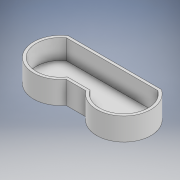
# Autodesk Inventor part: paitent remote box
Saved by Autodesk Inventor 2021 (Build 250183000, 183)
## iProperties
Created: 2023-01-12
Part Number: paitent remote box
Material: Generic
Document SubType Name: Modeling
Designer: boyle
Density: 1 g/cm^3
Appearance: Default
Author: boyle
Autodesk Inventor part; units mm, degrees
ref_plane "YZ Plane" through (0, 0, 0) normal (1, 0, 0) x (0, 1, 0)
ref_plane "XZ Plane" through (0, 0, 0) normal (0, 1, 0) x (-1, 0, 0)
ref_plane "XY Plane" through (0, 0, 0) normal (0, 0, 1) x (1, 0, 0)
sketch "Sketch1" plane through (0, 0, 0) normal (0, 1, 0) x (-1, 0, 0)
  line L0 (-23.3466, 0) -> (-154.4106, 0)
  line L1 (-102.87, 54.61) -> (-74.9238, 54.61)
  line L2 (-88.9, 0) -> (-23.3466, 0)
  line L3 (-88.9, 0) -> (-154.4106, 0)
  arc A0 (-102.87, 54.61) -> (-154.4106, 0) centre (-133.35, 31.75) ccw
  arc A1 (-23.3466, 0) -> (-74.9238, 54.61) centre (-44.4805, 31.7012) ccw
  point P0 (0, 0)
  dimension "d2" = 76.2
  dimension "d3" = 76.2
  dimension "d5" = 131.064
  dimension "d10" = 54.61
  constraints: 8 end point, 4 point on circle, 2 centre point, 2 collinear, 1 horizontal, 1 parallel, 1 point on line
  measures "d2" diameter of A0
  measures "d3" diameter of A1
  measures "d5" distance of L0.start L0.end
  measures "d10" distance between parallel lines of L1 L0
extrude "Extrusion1" add sketch "Sketch1" along normal blind 31.75
shell "Shell1" thickness 3.81 removed faces 1 at (84.227, 31.75, 18.2033)
body "Solid1"
